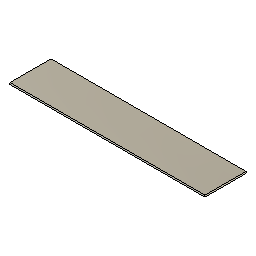
Back v6 (Autodesk Fusion 360 design; units mm, degrees)
Autodesk Fusion 360 part; units mm, degrees
sketch "Sketch1" plane through (0, 0, 0) normal (0, 0, 1) x (1, 0, 0)
  line L0 (108.5, 22.85) -> (-108.5, 22.85)
  line L1 (-108.5, 22.85) -> (-108.5, -22.85)
  line L2 (-108.5, -22.85) -> (108.5, -22.85)
  line L3 (108.5, -22.85) -> (108.5, 22.85)
  line L4 (108.5, 22.85) -> (-108.5, -22.85) construction
  line L5 (-108.5, 22.85) -> (108.5, -22.85) construction
  dimension "d1" = 217
  dimension "d2" = 45.7
  constraint horizontal L0
  constraint perpendicular L0 L1
  constraint parallel L0 L2
  constraint parallel L1 L3
  constraint coincident L4 origin
  constraint coincident L5 origin
  measures "d1" distance of L0.start L0.end
  measures "d2" distance of L0.end L1.end
extrude "Extrude1" add sketch "Sketch1" along normal blind 2
extrude "Extrude2" [suppressed]
extrude "Extrude3" [suppressed]
